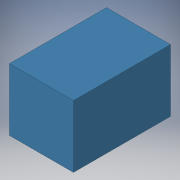
# Autodesk Inventor part: SmallBattery
Saved by Autodesk Inventor 2019 (Build 230136000, 136)
## iProperties
Created: 2018-03-28
Part Number: SmallBattery
Material: Generic
Document SubType Name: Modeling
Designer: james
Density: 2.83063 g/cm^3
Appearance: Default(1)
Mass: 4150.37 g
Surface Area: 789.709 cm^2
Volume: 1466.23 cm^3
Author: james
Autodesk Inventor part; units mm, degrees
ref_plane "YZ Plane" through (0, 0, 0) normal (1, 0, 0) x (0, 1, 0)
ref_plane "XZ Plane" through (0, 0, 0) normal (0, 1, 0) x (-1, 0, 0)
ref_plane "XY Plane" through (0, 0, 0) normal (0, 0, 1) x (1, 0, 0)
sketch "Sketch1" plane through (0, 0, 0) normal (0, 1, 0) x (-1, 0, 0)
  line L0 (37.7586, 60.4837) -> (-62.0634, 60.4837)
  line L1 (-62.0634, 60.4837) -> (-62.0634, -90.9003)
  line L2 (-62.0634, -90.9003) -> (37.7586, -90.9003)
  line L3 (37.7586, -90.9003) -> (37.7586, 60.4837)
  point P0 (0, 0)
  dimension "d0" = 151.384
  dimension "d1" = 99.822
  constraints: 8 end point, 2 parallel, 1 horizontal, 1 perpendicular
  measures "d0" distance of L2.end L0.start
  measures "d1" distance of L0.start L0.end
extrude "Extrusion1" add sketch "Sketch1" along normal blind 97.028
body "Solid1"
